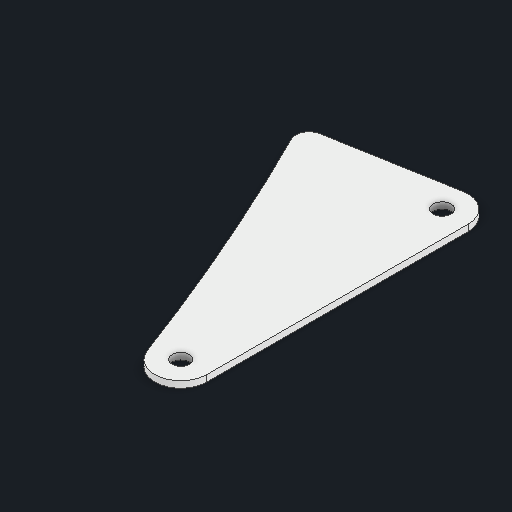
# Autodesk Inventor part: Magazine Gusset
Saved by Autodesk Inventor 2025.1 (Build 291241000, 241)
## iProperties
Created: 2024-12-31
Part Number: Magazine Gusset
Material: Acetal Resin, White
Document SubType Name: Modeling
Designer: Averey Ku
Density: 1.425 g/cm^3
Appearance: Smooth - White
Author: Averey Ku
Autodesk Inventor part; units mm, degrees
ref_plane "YZ Plane" through (0, 0, 0) normal (1, 0, 0) x (0, 1, 0)
ref_plane "XZ Plane" through (0, 0, 0) normal (0, 1, 0) x (-1, 0, 0)
ref_plane "XY Plane" through (0, 0, 0) normal (0, 0, 1) x (1, 0, 0)
sketch "main" plane through (0, 0, 0) normal (0, 0, 1) x (1, 0, 0)
  circle A0 centre (31.4944, -42.9627) radius 2.1844
  arc A1 (31.4944, -49.3127) -> (37.7453, -41.8453) centre (31.4944, -42.9627) ccw
  arc A2 (-34.2347, -37.0168) -> (-32.0056, -49.3127) centre (-32.0056, -42.9627) ccw
  arc A3 (-34.2347, -37.0168) -> (27.8848, -9.8628) centre (-257.1487, 557.5708) ccw
  line L0 (37.7453, -41.8453) -> (32.4355, -12.1413)
  line L1 (-32.0056, -49.3127) -> (31.4944, -49.3127)
  arc A4 (32.4355, -12.1413) -> (27.8848, -9.8628) centre (29.31, -12.7) ccw
  circle A5 centre (-32.0056, -42.9627) radius 2.0955
  point P0 (5.1717, -33.3366)
  point P1 (31.6842, -7.9384)
  dimension "d0" = 1270
  dimension "d1" = 12.7
  dimension "d2" = 12.7
  dimension "d3" = 3.175
  dimension "d4" = 4.191
  measures "d0" diameter of A3
  measures "d1" diameter of A2
  measures "d2" diameter of A1
  measures "d3" radius of A4
  measures "d4" diameter of A5
sketch "Sketch1" plane through (0, 0, 0) normal (0, 1, 0) x (-1, 0, 0)
  circle A0 centre (-0.1035, -63.4999) radius 2.1844
  arc A1 (-6.4535, -63.4896) -> (1.0037, -69.7526) centre (-0.1035, -63.4999) ccw
  arc A2 (5.9495, 2.2194) -> (-6.35, 0.0103) centre (0, 0) ccw
  arc A3 (5.9495, 2.2194) -> (33.0022, -59.9443) centre (600.8995, 224.1642) ccw
  line L0 (1.0037, -69.7526) -> (30.7163, -64.4912)
  line L1 (-6.35, 0.0103) -> (-6.4535, -63.4896)
  arc A4 (30.7163, -64.4912) -> (33.0022, -59.9443) centre (30.1627, -61.3648) ccw
  circle A5 centre (0, 0) radius 2.0955
  point P0 (0, 0)
  constraints: 1 other
extrude "Extrusion1" add sketch "Sketch1" along normal blind 1.5875
body "Solid1"
